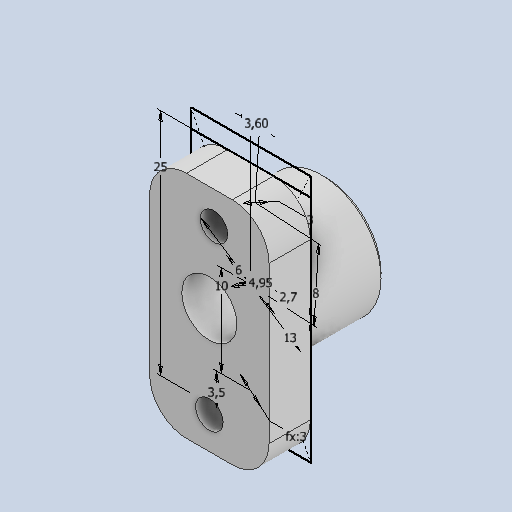
# Autodesk Inventor part: daVinci_Tool_Clutch
Saved by Autodesk Inventor 2024 (Build 280153000, 153)
## iProperties
Created: 2022-08-12
Part Number: daVinci_Tool_Clutch
Material: Generisch
Document SubType Name: Modeling
Designer: alexw
Density: 1 g/cm^3
Appearance: Vorgabe
Mass: 2.17984 g
Surface Area: 14.8905 cm^2
Volume: 2.17984 cm^3
Author: alexw
Autodesk Inventor part; units mm, degrees
ref_plane "YZ Plane" through (0, 0, 0) normal (1, 0, 0) x (0, 1, 0)
ref_plane "XZ Plane" through (0, 0, 0) normal (0, 1, 0) x (-1, 0, 0)
ref_plane "XY Plane" through (0, 0, 0) normal (0, 0, 1) x (1, 0, 0)
sketch "Skizze1" plane through (0, 0, 0) normal (0, 0, 1) x (1, 0, 0)
  line L0 (-6.5, 13.5) -> (6.5, 13.5)
  line L1 (6.5, 13.5) -> (6.5, -13.5)
  line L2 (6.5, -13.5) -> (-6.5, -13.5)
  line L3 (-6.5, -13.5) -> (-6.5, 13.5)
  line L4 (-6.5, 13.5) -> (6.5, -13.5) construction
  line L5 (6.5, 13.5) -> (-6.5, -13.5) construction
  line L6 (0, 0) -> (0.502324, 7.984214) construction
  line L7 (0, 0) -> (0, -13.5) construction
  circle A0 centre (0, -10) radius 1.5
  circle A1 centre (0.502324, 7.984214) radius 1.5
  line L8 (-6.5, 11.5) -> (6.5, 11.5)
  circle A2 centre (0, 0) radius 6.5
  circle A3 centre (0, 0) radius 2.475
  circle A4 centre (0, 0) radius 1.35
  circle A5 centre (0, 0) radius 3
  dimension "d13" = 3
  dimension "d14" = 3
  dimension "d15" = 3.5
  dimension "d16" = 10
  dimension "d17" = 8
  dimension "d18" = 3.6
  dimension "d23" = 4.95
  dimension "d26" = 2.7
  dimension "d29" = 6
  dimension "d37" = 13
  dimension "d39" = 25
  constraints: 18 end point, 6 centre point, 5 coincident, 3 midpoint, 3 point on line, 2 parallel, 2 perpendicular, 1 horizontal, 1 tangent
  measures "d13" diameter of A1
  measures "d14" diameter of A0
  measures "d15" distance from line of A0.centre L2
  measures "d16" distance of L6.start A0.centre
  measures "d17" distance of L6.start L6.end
  measures "d18" angle of L7 L6
  measures "d23" diameter of A3
  measures "d26" diameter of A4
  measures "d29" diameter of A5
  measures "d37" diameter of A2
  measures "d39" distance between parallel lines of L8 L2
extrude "Extrusion1" add sketch "Skizze1" along normal blind 4.5 contours L8 L1 A2 L3 | A2 L1 L2 L3 | A2 | A3 | A4 | A5
extrude "Extrusion2" add sketch "Skizze1" against normal blind 8.2 contours A2 | A5
extrude "Extrusion3" cut sketch "Skizze1" along normal through all contours A4
extrude "Extrusion4" cut sketch "Skizze1" against normal blind 7 from surface at 4.5 contours A3 | A4 | A5
chamfer "Fase1" distance 0.5 angle 45 1 edges at (-6.5, 0, -8.2)
fillet "Rundung1" radius 4 4 edges at (6.5, 11.5, 2.25) (-6.5, 11.5, 2.25) (6.5, -13.5, 2.25) (-6.5, -13.5, 2.25)
extrude "Extrusion6" add sketch "Skizze1" against normal blind 4.95 contours A3 | A5
extrude "Extrusion7" cut sketch "Skizze1" against normal blind 1 contours A3 | A5
equation "\"d14\" = d13"
